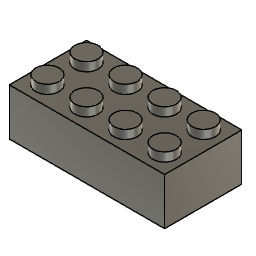
lego_brick v1 (Autodesk Fusion 360 design; units mm, degrees)
Autodesk Fusion 360 part; units mm, degrees
sketch "Sketch1" plane through (0, 0, 0) normal (0, 0, 1) x (1, 0, 0)
  line L0 (0, 0) -> (31.8, 0)
  line L1 (31.8, 0) -> (31.8, 15.8)
  line L2 (31.8, 15.8) -> (0, 15.8)
  line L3 (0, 15.8) -> (0, 0)
  dimension "d1" = 31.8
  dimension "d2" = 15.8
  constraint horizontal L0
  constraint vertical L1
  constraint horizontal L2
  constraint vertical L3
  constraint coincident L0.start L3.end
  measures "d1" distance of L0.start L0.end
  measures "d2" distance of L0.start L2.end
extrude "Extrude1" add sketch "Sketch1" along normal blind 9.6
sketch "Sketch2" plane through (0, 0, 0) normal (0, 1, 0) x (1, 0, 0)
shell "Shell1" thickness 1 removed faces 1 at (21.2, 5.2667, 0)
sketch "Sketch3" plane through (0, 0, 9.6) normal (0, 0, 1) x (-1, 0, 0)
  line L0 (0, -15.8) -> (0, 0)
  line L1 (0, 0) -> (-31.8, 0)
  line L2 (-31.8, 0) -> (-31.8, -15.8)
  line L3 (-31.8, -15.8) -> (0, -15.8)
  circle A0 centre (-3.9, -11.9) radius 2.4
  circle A1 centre (-11.9, -11.9) radius 2.4
  circle A2 centre (-19.9, -11.9) radius 2.4
  circle A3 centre (-27.9, -11.9) radius 2.4
  circle A4 centre (-3.9, -3.9) radius 2.4
  circle A5 centre (-11.9, -3.9) radius 2.4
  circle A6 centre (-19.9, -3.9) radius 2.4
  circle A7 centre (-27.9, -3.9) radius 2.4
  dimension "d6" = 4.8
  dimension "d7" = 3.9
  dimension "d8" = 3.9
  dimension "d11" = -8
  dimension "d12" = 8
  measures "d6" diameter of A0
  measures "d7" distance of L3 A0.centre
  measures "d8" distance of L0 A0.centre
extrude "Extrude2" add sketch "Sketch3" along normal blind 1.8 contours A0 | A1 | A2 | A3 | A4 | A5 | A6 | A7
sketch "Sketch4" plane through (0, 0, 8.6) normal (0, 0, -1) x (1, 0, 0)
  line L0 (1, -1) -> (1, -14.8)
  line L1 (1, -14.8) -> (30.8, -14.8)
  line L2 (30.8, -14.8) -> (30.8, -1)
  line L3 (30.8, -1) -> (1, -1)
  circle A0 centre (3.9, -3.9) radius 1.3
  circle A1 centre (3.9, -3.9) radius 2.4
  line L4 (0, 0) -> (31.8, 0)
  line L5 (0, -15.8) -> (0, 0)
  circle A2 centre (11.9, -3.9) radius 1.3
  circle A3 centre (19.9, -3.9) radius 1.3
  circle A4 centre (27.9, -3.9) radius 1.3
  circle A5 centre (3.9, -11.9) radius 1.3
  circle A6 centre (11.9, -11.9) radius 1.3
  circle A7 centre (19.9, -11.9) radius 1.3
  circle A8 centre (27.9, -11.9) radius 1.3
  dimension "d15" = 2.6
  dimension "d16" = 3.9
  dimension "d17" = 3.9
  dimension "d20" = 8
  dimension "d21" = -8
  constraint concentric A0 A1
  measures "d15" diameter of A0
  measures "d16" distance of A0.centre L4
  measures "d17" distance of A0.centre L5
extrude "Extrude3" cut sketch "Sketch4" against normal blind 1.7 contours A0 | A2 | A3 | A4 | A5 | A6 | A7 | A8
sketch "Sketch5" plane through (0, 0, 8.6) normal (0, 0, -1) x (1, 0, 0)
  circle A0 centre (11.9, -11.9) radius 1.3
  circle A1 centre (19.9, -3.9) radius 1.3
  circle A2 centre (11.9, -3.9) radius 1.3
  circle A3 centre (19.9, -11.9) radius 1.3
  circle A4 centre (3.9, -11.9) radius 1.3
  circle A5 centre (27.9, -3.9) radius 1.3
  circle A6 centre (3.9, -3.9) radius 1.3
  circle A7 centre (27.9, -11.9) radius 1.3
  line L0 (1, -1) -> (1, -14.8)
  line L1 (1, -14.8) -> (30.8, -14.8)
  line L2 (30.8, -14.8) -> (30.8, -1)
  line L3 (30.8, -1) -> (1, -1)
  circle A8 centre (7.9, -7.9) radius 2.4
  line L4 (0, -15.8) -> (0, 0)
  line L5 (31.8, -15.8) -> (0, -15.8)
  circle A9 centre (7.9, -7.9) radius 3.255
  circle A10 centre (15.9, -7.9) radius 2.4
  circle A11 centre (15.9, -7.9) radius 3.255
  circle A12 centre (23.9, -7.9) radius 2.4
  circle A13 centre (23.9, -7.9) radius 3.255
  dimension "d24" = 4.8
  dimension "d25" = 7.9
  dimension "d26" = 7.9
  dimension "d27" = 6.51
  dimension "d30" = 8
  dimension "d31" = 0
  constraint concentric A8 A9
  measures "d24" diameter of A8
  measures "d25" distance of A8.centre L4
  measures "d26" distance of A8.centre L5
  measures "d27" diameter of A9
extrude "Extrude4" add sketch "Sketch5" along normal blind 8.6 contours A9 | A11 | A13
sketch "Sketch6" plane through (0, 0, 0) normal (0, 0, -1) x (1, 0, 0)
  circle A0 centre (15.9, -7.9) radius 2.4
  circle A1 centre (15.9, -7.9) radius 3.255
  line L0 (1, -1) -> (30.8, -1)
  line L1 (30.8, -14.8) -> (1, -14.8)
  line L2 (15.9, -1) -> (15.9, -4.645) construction
  line L3 (15.9, -11.155) -> (15.9, -14.8) construction
  line L4 (16.3, -1) -> (16.3, -4.6697)
  line L5 (16.3, -11.1303) -> (16.3, -14.8)
  line L6 (15.5, -1) -> (15.5, -4.6697)
  line L7 (15.5, -11.1303) -> (15.5, -14.8)
  constraint midpoint L0 L2.start
  constraint midpoint L1 L3.end
  constraint coincident A1 L2.end
  constraint collinear L2 L3
  constraint coincident A1 L4.end
  constraint collinear L4 L5
  constraint coincident A1 L6.end
  constraint collinear L6 L7
  constraint coincident A1 L3.start
  constraint coincident A1 L5.start
  constraint coincident A1 L7.start
extrude "Extrude5" add sketch "Sketch6" against normal blind 8.6 contours A1 L0 L4 L6 | A1 L1 L5 L7
sketch "Sketch7" plane through (0, 15.8, 0) normal (0, 1, 0) x (-1, 0, 0)
  line L0 (-31.8, 0) -> (0, 0)
  line L1 (0, 0) -> (0, 9.6)
  line L2 (0, 9.6) -> (-31.8, 9.6)
  line L3 (-31.8, 9.6) -> (-31.8, 0)
  line L4 (-30.1253, 3.1841) -> (-0.9632, 3.1841) construction
  line L5 (-0.9632, 3.1841) -> (-0.9632, 7.1841) construction
  line L6 (-0.9632, 7.1841) -> (-30.1253, 7.1841) construction
  line L7 (-30.1253, 7.1841) -> (-30.1253, 3.1841) construction
  text T0 "IoT BOOTCAMP" font "Arial" height 4 align ink ink in box 0 x 0 at (-30.1253, 3.1841) x (1, 0) y (0, 1) spacing 1 kerned height is em
  constraint perpendicular L4 L5
  constraint parallel L4 L6
  constraint parallel L5 L7
extrude "Extrude6" add sketch "Sketch7" along normal blind 1 text T0
